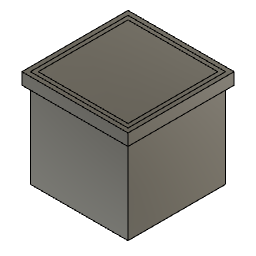
box (Autodesk Fusion 360 design; units mm, degrees)
Autodesk Fusion 360 part; units mm, degrees
sketch "Sketch1" plane through (0, 0, 0) normal (0, 0, 1) x (1, 0, 0)
  line L0 (25, -25) -> (-25, -25)
  line L1 (-25, -25) -> (-25, 25)
  line L2 (-25, 25) -> (25, 25)
  line L3 (25, 25) -> (25, -25)
  line L4 (25, -25) -> (-25, 25) construction
  line L5 (-25, -25) -> (25, 25) construction
  dimension "d1" = 50
  dimension "d2" = 50
  constraint horizontal L0
  constraint perpendicular L0 L1
  constraint parallel L0 L2
  constraint parallel L1 L3
  constraint coincident L4 origin
  constraint coincident L5 origin
  measures "d1" distance of L0.end L1.end
  measures "d2" distance of L1.end L2.end
extrude "Extrude1" add sketch "Sketch1" along normal blind 50 makes body 1
shell "Shell1" thickness 2 removed faces 1 at (8.3333, -8.3333, 50) on bodies 1
sketch "Sketch3" plane through (0, 0, 50) normal (0, 0, 1) x (-1, 0, 0)
  line L0 (-23, -23) -> (-23, 23)
  line L1 (-23, 23) -> (23, 23)
  line L2 (23, 23) -> (23, -23)
  line L3 (23, -23) -> (-23, -23)
  line L4 (-25, -25) -> (25, -25)
  line L5 (25, -25) -> (25, 25)
  line L6 (25, 25) -> (-25, 25)
  line L7 (-25, 25) -> (-25, -25)
  line L8 (-25, -25) -> (-25, 25) construction
  line L9 (-25, 25) -> (25, 25) construction
  line L10 (25, 25) -> (25, -25) construction
  line L11 (25, -25) -> (-25, -25) construction
  line L12 (27.2, 27.2) -> (27.2, -27.2)
  line L13 (27.2, -27.2) -> (-27.2, -27.2)
  line L14 (-27.2, -27.2) -> (-27.2, 27.2)
  line L15 (-27.2, 27.2) -> (27.2, 27.2)
  dimension "d10" = -2.2
extrude "Extrude3" add sketch "Sketch3" against normal blind 6 separate body contours L0 L1 L2 L3 | L4 L5 L6 L7 | L12 L13 L14 L15 makes body 2
shell "Shell3" thickness 2 removed faces 1 at (-9.0667, 9.0667, 44) on bodies 2
sketch "Sketch2" plane through (0, 0, 50) normal (0, 0, 1) x (-1, 0, 0)
  line L0 (27.2, -27.2) -> (-27.2, -27.2)
  line L1 (-27.2, -27.2) -> (-27.2, 27.2)
  line L2 (-27.2, 27.2) -> (27.2, 27.2)
  line L3 (27.2, 27.2) -> (27.2, -27.2)
extrude "Extrude2" [rolled back] along distance -6 taper angle 0
shell "Shell2" [rolled back] inner thickness 2
move_body "Move1" [rolled back]
equation "d10 = -( 2 mm + 0.2 mm )"
